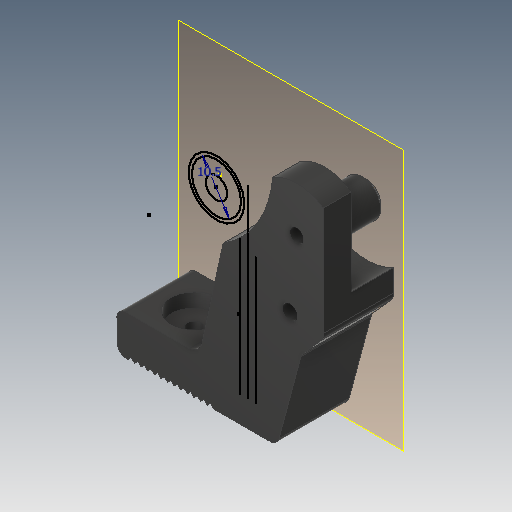
# Autodesk Inventor part: Extruder Arm
Saved by Autodesk Inventor 2017 (Build 210142000, 142)
## iProperties
Created: 2016-06-27
Part Number: Extruder Arm
Material: Acetal Resin, Black
Document SubType Name: Modeling
Designer: joshmamo
Density: 1.425 g/cm^3
Appearance: Smooth - Black
Mass: 17.3159 g
Surface Area: 55.097 cm^2
Volume: 12.1515 cm^3
Author: joshmamo
Autodesk Inventor part; units mm, degrees
ref_plane "YZ Plane" through (0, 0, 0) normal (1, 0, 0) x (0, 1, 0)
ref_plane "XZ Plane" through (0, 0, 0) normal (0, 1, 0) x (-1, 0, 0)
ref_plane "XY Plane" through (0, 0, 0) normal (0, 0, 1) x (1, 0, 0)
ref_plane "Work Plane1" through (9.6095, -20.0425, -0.002) normal (0, 0, 1) x (0, -1, 0)
sketch "Sketch1" plane through (9.6095, -20.0425, -0.002) normal (0, 0, 1) x (0, -1, 0)
  line L0 (8.0789, 6.3305) -> (-15.1679, 27.0243)
  line L1 (0.3675, -1.0971) -> (0.3675, -14.5912)
  line L2 (2.8962, -16.5081) -> (6.3982, -16.5081)
  line L3 (8.9372, -13.9577) -> (8.9372, -12.9037)
  line L4 (-16.702, 27.52) -> (-40.068, 27.52)
  line L5 (-1.5025, 12.8896) -> (-5.5053, 12.8896)
  line L6 (0.348, 8.1669) -> (-3.0575, 8.1669)
  line L7 (8.9372, -13.9577) -> (34.426, -13.9577) construction
  line L8 (-4.0492, 17.1267) -> (8.0789, 6.3305)
  line L9 (8.0789, 6.3305) -> (-15.1679, 27.0243)
  line L10 (-38.656, 27.52) -> (-16.702, 27.52)
  line L11 (0.3675, -7.1533) -> (0.3675, -1.0971)
  line L12 (0.3675, -7.1533) -> (0.3675, -14.5912)
  line L13 (6.3982, -16.5081) -> (2.8962, -16.5081)
  line L14 (2.8962, -16.5081) -> (6.9382, -16.5081)
  line L15 (8.9372, -14.4977) -> (8.9372, -14.2263)
  arc A0 (6.9382, -16.5081) -> (8.9372, -14.4977) centre (6.9372, -14.5081) ccw
  arc A1 (0.3675, -14.5912) -> (2.8962, -16.5081) centre (2.3675, -14.5793) ccw
  arc A2 (8.9372, 4.6884) -> (8.0789, 6.3305) centre (6.9372, 4.6884) ccw
  arc A3 (-15.1679, 27.0243) -> (-16.702, 27.52) centre (-16.4977, 25.5305) ccw
  arc A4 (-19.5823, 16.2837) -> (-20.8514, 16.738) centre (-20.8514, 14.738) ccw
  arc A5 (-39.9409, 27.52) -> (-40.2505, 16.738) centre (-32.041, 21.8977) ccw
  circle A6 centre (-17.1179, 20.3803) radius 1.35
  circle A7 centre (-17.1179, 20.3803) radius 1.6
  line L16 (8.9372, 4.1585) -> (8.2301, 3.4514)
  line L17 (8.9372, 4.1585) -> (9.9372, 4.1585) construction
  line L18 (8.2301, 3.4514) -> (8.9372, 2.7443)
  line L19 (8.9372, 2.7443) -> (8.2301, 2.0372)
  line L20 (8.2301, 2.0372) -> (8.9372, 1.3301)
  line L21 (8.9372, 1.3301) -> (8.2301, 0.623)
  line L22 (8.2301, 0.623) -> (8.9372, -0.0841)
  line L23 (8.9372, -0.0841) -> (8.2301, -0.7912)
  line L24 (8.2301, -0.7912) -> (8.9372, -1.4983)
  line L25 (8.9372, -1.4983) -> (8.2301, -2.2054)
  line L26 (8.2301, -2.2054) -> (8.9372, -2.9125)
  line L27 (8.9372, -2.9125) -> (8.2301, -3.6197)
  line L28 (8.2301, -3.6197) -> (8.9372, -4.3268)
  line L29 (8.9372, -4.3268) -> (8.2301, -5.0339)
  line L30 (8.2301, -5.0339) -> (8.9372, -5.741)
  line L31 (8.9372, -5.741) -> (8.2301, -6.4481)
  line L32 (8.2301, -6.4481) -> (8.9372, -7.1552)
  line L33 (8.9372, -7.1552) -> (8.2301, -7.8623)
  line L34 (8.2301, -7.8623) -> (8.9372, -8.5694)
  line L35 (8.9372, -8.5694) -> (8.2301, -9.2765)
  line L36 (8.2301, -9.2765) -> (8.9372, -9.9836)
  line L37 (8.9372, -9.9836) -> (8.2301, -10.6907)
  line L38 (8.2301, -10.6907) -> (8.9372, -11.3978)
  line L39 (8.9372, -11.3978) -> (8.2301, -12.1049)
  line L40 (8.2301, -12.1049) -> (8.9372, -12.812)
  line L41 (8.9372, -12.812) -> (8.2301, -13.5191)
  line L42 (8.2301, -13.5191) -> (8.9372, -14.2263)
  line L43 (8.9372, -14.4977) -> (8.9372, -14.2263)
  line L44 (8.9372, 4.1585) -> (8.9372, 4.6884)
  circle A8 centre (-32.3465, 4.6135) radius 5.95
  line L45 (-1.5025, 1.4391) -> (-22.7599, 6.1599)
  arc A9 (-22.7599, 6.1599) -> (-40.2505, 16.738) centre (-42.147, -6.1471) ccw
  arc A10 (0.3675, -1.0971) -> (-1.5025, 1.4391) centre (-2.6051, -1.3314) ccw
  point P0 (-20.0425, -9.6095)
  point P1 (-21.046, 16.738)
  point P2 (0.3675, -14.5912)
  point P3 (8.0789, 6.3305)
  dimension "d1" = 2
  dimension "d2" = 2
  dimension "d4" = 3.2
  dimension "d5" = 1
  dimension "d6" = 135
  dimension "d7" = 1
  dimension "d8" = 1
  dimension "d9" = 1
  dimension "d10" = 1
  dimension "d11" = 1
  dimension "d12" = 1
  dimension "d13" = 1
  dimension "d14" = 1
  dimension "d15" = 1
  dimension "d16" = 1
  dimension "d17" = 1
  dimension "d18" = 1
  constraints: 97 end point, 18 point on circle, 11 centre point, 7 point on line, 1 coincident, 1 horizontal, 2 other
  measures "d1" radius of A0
  measures "d2" radius of A2
  measures "d4" diameter of A7
  measures "d5" distance of L16.start L16.end
  measures "d6" angle of L16 L17
  measures "d7" distance of L18.end L19.end
  measures "d8" distance of L20.end L21.end
  measures "d9" distance of L22.end L23.end
  measures "d10" distance of L24.end L25.end
  measures "d11" distance of L26.end L27.end
  measures "d12" distance of L28.end L29.end
  measures "d13" distance of L30.end L31.end
  measures "d14" distance of L32.end L33.end
  measures "d15" distance of L34.end L35.end
  measures "d16" distance of L36.end L37.end
  measures "d17" distance of L38.end L39.end
  measures "d18" distance of L40.end L41.end
extrude "Extrusion1" add sketch "Sketch1" along normal blind 15 contours A2 L44 L16 L18 L19 L20 L21 L22 L23 L24 L25 L26 L27 L28 L29 L30 L31 L32 L33 L34 L35 L36 L37 L38 L39 L40 L41 L42 L15 A0 L14 L2 A1 L1 A10 L45 A9 A5 L4 A3 L0
sketch "Sketch2" plane through (9.6095, -20.0425, -0.002) normal (0, 0, -1) x (-1, 0, 0)
  point P0 (9.6095, 20.0425)
sketch "Sketch3" plane through (9.6095, -20.0425, -0.002) normal (0, 0, -1) x (-1, 0, 0)
  circle A0 centre (-21.8558, 31.9836) radius 3.4745 projected
  circle A1 centre (-21.8558, 31.9836) radius 12
  circle A2 centre (-21.8558, 31.9836) radius 3.95
  point P0 (9.6095, 20.0425)
  dimension "d21" = 24
  dimension "d22" = 7.9
  constraints: 2 centre point, 2 coincident
  measures "d21" diameter of A1
  measures "d22" diameter of A2
extrude "Extrusion2" cut sketch "Sketch3" against normal blind 9 contours A1
chamfer "Chamfer1" distance 1 angle 45 1 edges at (35.4153, 11.9411, -0.002)
sketch "Sketch4" plane through (9.6095, -20.0425, -0.002) normal (0, 0, -1) x (-1, 0, 0)
  line L0 (-4.1585, -8.9372) -> (-4.6884, -8.9372) projected
  line L1 (-4.6884, -8.9372) -> (-16.1537, -8.9372)
  line L2 (-4.6884, -8.9372) -> (6.777, -8.9372) construction
  line L3 (-18.0856, -7.4548) -> (-22.9084, 10.5443)
  line L4 (-6.3305, -8.0789) -> (-27.0243, 15.1679) projected
  line L5 (-26.876, 15.012) -> (-6.32, -8.08) projected
  arc A0 (-6.3305, -8.0789) -> (-4.6884, -8.9372) centre (-4.6884, -6.9372) ccw projected
  arc A1 (-18.0856, -7.4548) -> (-16.1537, -8.9372) centre (-16.1537, -6.9372) ccw
  line L6 (-12.8978, 2.9391) -> (-8.1342, 2.9391)
  line L7 (-10.516, 2.9391) -> (-10.516, -9.4975)
  point P0 (9.6095, 20.0425)
  point P1 (-17.6884, -8.9372)
  point P2 (-6.1599, -8.2598)
  point P3 (-27.0243, 15.1679)
  dimension "d28" = 13
  dimension "d29" = 180
  dimension "d30" = 105
  dimension "d31" = 2
  constraints: 10 end point, 3 horizontal, 2 point on circle, 2 point on line, 2 tangent, 1 centre point, 1 collinear, 1 midpoint, 1 vertical, 3 other
  measures "d28" distance of L0.end point (-17.688, -8.937)
  measures "d29" angle of L2 L1
  measures "d30" angle of L1 L3
  measures "d31" radius of A1
extrude "Extrusion3" add sketch "Sketch4" against normal up to surface (15 mm away)
fillet "Fillet1" radius 2 1 edges at (32.5179, -9.4982, 7.498)
sketch "Sketch5" plane through (13.768, -28.9797, -0.002) normal (0, -1, 0) x (1, 0, 0)
  line L0 (8.7614, -11.1681) -> (8.7614, 10.6543)
  line L1 (4.0052, -11.1681) -> (4.0052, 10.6543)
  line L2 (8.7614, -0.5012) -> (8.7614, 4.1988)
  line L3 (12.1475, 0) -> (12.1475, 15)
  line L4 (8.7614, 0.9988) -> (13.4614, 0.9988) construction
  line L5 (8.7614, 4.1988) -> (7.8182, 4.1988)
  line L6 (8.7614, 4.1988) -> (8.7614, 5.6988)
  line L7 (8.7614, 5.6988) -> (7.2614, 5.6988)
  arc A0 (7.2614, 4.0988) -> (7.2614, 7.2988) centre (7.2614, 5.6988) ccw
  line L8 (4.0052, 5.6988) -> (5.5052, 5.6988)
  arc A1 (5.5052, 7.2988) -> (5.5052, 4.0988) centre (5.5052, 5.6988) ccw
  line L9 (5.5052, 4.0988) -> (7.2614, 4.0988)
  line L10 (7.2614, 7.2988) -> (5.5052, 7.2988)
  circle A2 centre (6.3833, 5.6988) radius 4.5
  point P0 (-13.768, 0.002)
  dimension "d35" = 4.7
  dimension "d36" = 90
  dimension "d37" = 1.5
  dimension "d38" = 1.5
  dimension "d39" = 3.2
  dimension "d40" = 1.5
  dimension "d41" = 3.2
  dimension "d42" = 9
  constraints: 22 end point, 5 point on circle, 3 centre point, 3 point on line, 2 coincident
  measures "d35" distance of L2.start L2.end
  measures "d36" angle of L4 L2
  measures "d37" distance of L2.end L6.end
  measures "d38" distance of L6.end L7.end
  measures "d39" diameter of A0
  measures "d40" distance of L8.start L8.end
  measures "d41" diameter of A1
  measures "d42" diameter of A2
extrude "Extrusion4" cut sketch "Sketch5" against normal through all contours A0 L9 A1 L1 L10 L0 | L0 A0 | A1 L1
sketch "Sketch6" plane through (13.768, -28.9797, -0.002) normal (0, -1, 0) x (1, 0, 0)
  line L0 (7.2614, 4.0988) -> (5.5052, 4.0988) projected
  line L1 (5.5052, 7.2988) -> (7.2614, 7.2988) projected
  line L2 (6.3833, 7.2988) -> (6.3833, 4.0988)
  circle A0 centre (6.3833, 5.6988) radius 4.5
  point P0 (-13.768, 0.002)
  dimension "d45" = 9
  constraints: 3 midpoint, 2 end point, 1 centre point
  measures "d45" diameter of A0
extrude "Extrusion5" cut sketch "Sketch6" against normal blind 5.7
sketch "Sketch7" plane through (-4.9817, -20.41, -0.002) normal (0, 1, 0) x (1, 0, 0)
  line L0 (12.0753, 7.6947) -> (12.0753, -8.3858)
  line L1 (12.0753, 7.6947) -> (28.1558, 7.6947) construction
  line L2 (12.0753, -8.3858) -> (2.0753, -8.3858)
  line L3 (2.4862, 0) -> (2.4862, -15) projected
  line L4 (7.0753, -8.3858) -> (7.0753, 0)
  line L5 (7.0753, 0) -> (7.0753, -15)
  circle A0 centre (7.0753, -7.5) radius 1.6
  circle A1 centre (7.0753, -7.5) radius 5
  point P0 (4.9817, -0.002)
  dimension "d48" = 90
  dimension "d49" = 10
  dimension "d50" = 90
  dimension "d51" = 0
  dimension "d52" = 3.2
  constraints: 10 end point, 2 centre point, 2 midpoint, 2 perpendicular, 1 coincident, 1 horizontal, 1 tangent, 1 vertical
  measures "d48" angle of L0 L1
  measures "d49" distance of L0.end L2.end
  measures "d50" angle of L0 L2
  measures "d51" distance between parallel lines of L5 L4
  measures "d52" diameter of A0
extrude "Extrusion6" cut sketch "Sketch7" against normal blind 3 contours A1 L2 A0 L4 | L4 A0 L2 L3 A1 | A1 L5 A0 L2 | L3 L2 A1 | A1 L3 L2 A0 L5 | L3 A1 L2
sketch "Sketch8" plane through (2.0937, -20.41, 7.498) normal (0, 1, 0) x (1, 0, 0)
  circle A0 centre (0, 0) radius 1.6 projected
  circle A1 centre (0, 0) radius 1.6 projected
  point P0 (-2.0937, 7.498)
extrude "Extrusion7" cut sketch "Sketch8" against normal through all
sketch "Sketch9" plane through (9.6095, -20.0425, 14.998) normal (0, 0, 1) x (1, 0, 0)
  circle A0 centre (4.6135, 32.3465) radius 5.95
  line L0 (13.0199, -3.2372) -> (13.0199, 23.864)
  line L1 (9.6638, -3.2372) -> (9.6638, 25.4935)
  line L2 (11.4199, -3.2372) -> (11.4199, 26.0597)
  line L3 (11.3976, 13.6313) -> (11.3976, 36.2153)
  circle A1 centre (4.6135, 32.3465) radius 2.3
  circle A2 centre (4.6135, 32.3465) radius 5.25
  point P0 (-9.6095, 20.0425)
  point P1 (9.6415, 11.4924)
  point P2 (11.4199, 26.0597)
  dimension "d57" = 10.5
  constraints: 4 end point, 3 centre point, 1 coincident, 6 other
  measures "d57" diameter of A2
fillet "Fillet2" radius 1 6 edges at (20.8112, 6.4192, 7.2968) (20.8112, 6.4192, 4.0968) (22.5633, 3.894, 6.1518) (19.9553, 6.1262, 4.0968) (19.9553, 6.1262, 7.2968) (17.6732, 4.0664, 5.6968)
sketch "Sketch10" plane through (31.4653, 11.9411, -0.002) normal (0, 0, -1) x (-1, 0, 0)
  circle A0 centre (0, 0) radius 1.5
  point P0 (31.4653, -11.9411)
  dimension "d59" = 3
  constraints: 1 centre point
  measures "d59" diameter of A0
extrude "Extrusion8" cut sketch "Sketch10" against normal through all
body "Solid1"
